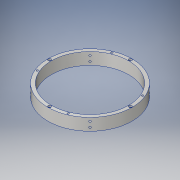
# Autodesk Inventor part: ontelMounting
Saved by Autodesk Inventor 2016 SP1 (Build 200210100, 210)
## iProperties
Created: 2015-12-10
Part Number: ontelMounting
Material: Aluminum 6061
Document SubType Name: Modeling
Designer: Dave
Density: 2.7 g/cm^3
Appearance: Aluminum - Flat
Mass: 1717.63 g
Surface Area: 1312.48 cm^2
Volume: 636.161 cm^3
Author: Dave
Autodesk Inventor part; units mm, degrees
ref_plane "YZ Plane" through (0, 0, 0) normal (1, 0, 0) x (0, 1, 0)
ref_plane "XZ Plane" through (0, 0, 0) normal (0, 1, 0) x (-1, 0, 0)
sketch "Sketch1" plane through (0, 0, 0) normal (0, 1, 0) x (-1, 0, 0)
  circle A0 centre (0, 0) radius 155.575
  circle A1 centre (0, 0) radius 142.875
  dimension "d0" = 311.15
  dimension "d1" = 12.7
  constraints: 2 centre point, 1 coincident
  measures "d0" diameter of A0
  measures "d1" radial gap between concentric circles of A1 A0
extrude "Extrusion1" add sketch "Sketch1" along normal blind 44.45
sketch "Sketch2" plane through (0, 44.45, 0) normal (0, 1, 0) x (1, 0, 0)
  circle A0 centre (0, -149.225) radius 3.8282
  point P0 (0, 0)
  dimension "d4" = 149.225
  constraints: 1 centre point
  measures "d4" distance of A0.centre point (0, 0)
hole "Hole1" at (0, 44.45, 149.225) direction (0, -1, 0) diameter 6.7564 end through all counterbore diameter 11.1252 counterbore depth 6.35 clearance for "Socket Head Cap Screw" size "1/4" standard "Ansi Unified Screw Threads"
pattern_circular "Circular Pattern1" count 4 over 360 about axis through (0, -10, 0) along (0, 1, 0) of "Hole1"
sketch "Sketch3" plane through (0, 44.45, 0) normal (0, 1, 0) x (1, 0, 0)
  line L0 (0, 0) -> (-167.6109, 167.6109) construction
  line L1 (0, 0) -> (237.0376, 0) construction
  circle A0 centre (0, 0) radius 155.575 projected
  point P0 (-110.0081, 110.0081)
  dimension "d15" = 135
  constraints: 4 end point, 1 equal length, 1 horizontal, 1 point on line, 2 other
  measures "d15" angle of L1 L0
ref_plane "Work Plane1" through (-110.0081, 44.45, -110.0081) normal (-0.7071, 0, -0.7071) x (0, -1, 0)
sketch "Sketch4" plane through (-110.0081, 44.45, -110.0081) normal (-0.7071, 0, -0.7071) x (0, -1, 0)
  circle A0 centre (12.7, 0) radius 2.9411
  circle A1 centre (31.75, 0) radius 3.3282
  line L0 (0, 155.575) -> (0, -155.575) projected
  point P0 (44.45, 0)
  dimension "d16" = 12.7
  dimension "d17" = 19.05
  constraints: 2 centre point
  measures "d16" distance from line of A0.centre L0
  measures "d17" distance of A1.centre A0.centre
hole "Hole2" at (-110.0081, 12.7, -110.0081) at (-110.0081, 31.75, -110.0081) direction (0.7071, 0, 0.7071) diameter 6.5278 end through all clearance for "Flat Head Machine Screw (82)" size "1/4" standard "Ansi Unified Screw Threads"
pattern_circular "Circular Pattern2" count 4 over 360 about axis through (0, -10, 0) along (0, 1, 0) of "Hole2"
sketch "Sketch5" plane through (0, 44.45, 0) normal (0, 1, 0) x (1, 0, 0)
  line L0 (0, 0) -> (137.8659, 57.1059) construction
  line L1 (0, 0) -> (149.225, 0) construction
  circle A0 centre (137.8659, 57.1059) radius 3.2687
  dimension "d28" = 149.225
  dimension "d29" = 22.5
  constraints: 4 end point, 1 centre point, 1 coincident, 1 equal length, 1 horizontal
  measures "d28" distance of L0.start L0.end
  measures "d29" angle of L1 L0
hole "Hole3" at (137.8659, 44.45, -57.1059) direction (0, -1, 0) diameter 6.7564 end through all clearance for "Flat Head Machine Screw (82)" size "1/4" standard "Ansi Unified Screw Threads"
pattern_circular "Circular Pattern3" count 4 over 360 about axis through (0, 0, 0) along (0, 1, 0) of "Hole3"
equation "\"d0\" = width + 2 * radiusCtr"
equation "\"d1\" = width"
equation "\"d4\" = radiusCtr"
equation "\"d28\" = radiusCtr"
equation "\"radiusCtr\" = 149.225"
equation "\"width\" = 12.7"
body "Solid1"
